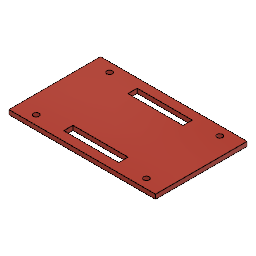
Nikon Labophot - Power supply fixation v2 (Autodesk Fusion 360 design; units mm, degrees)
Autodesk Fusion 360 part; units mm, degrees
sketch "sketch 283" plane through (0, 8, 0) normal (0, 1, 0) x (-1, 0, 0)
  line L0 (0, 82) -> (30, 82)
  line L1 (30, 82) -> (30, 77)
  line L2 (30, 77) -> (0, 77)
  line L3 (0, 77) -> (0, 82)
  circle A0 centre (45, 82) radius 1.5
  circle A1 centre (45, 42) radius 1.5
  circle A2 centre (-15, 82) radius 1.5
  line L4 (0, 47) -> (30, 47)
  line L5 (30, 47) -> (30, 42)
  line L6 (30, 42) -> (0, 42)
  line L7 (0, 42) -> (0, 47)
  circle A3 centre (-15, 42) radius 1.5
  line L8 (-25, 87) -> (55, 87)
  line L9 (-25, 37) -> (-25, 87)
  line L10 (55, 37) -> (-25, 37)
  line L11 (55, 87) -> (55, 37)
extrude "Extrude1" add sketch "sketch 283" along normal blind 2.5
